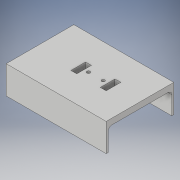
# Autodesk Inventor part: breadBoardMt
Saved by Autodesk Inventor 2019 (Build 230136000, 136)
## iProperties
Created: 2019-10-26
Part Number: breadBoardMt
Material: Generic
Document SubType Name: Modeling
Designer: test
Density: 1 g/cm^3
Appearance: Default
Author: test
Autodesk Inventor part; units mm, degrees
ref_plane "YZ Plane" through (0, 0, 0) normal (1, 0, 0) x (0, 1, 0)
ref_plane "XZ Plane" through (0, 0, 0) normal (0, 1, 0) x (-1, 0, 0)
ref_plane "XY Plane" through (0, 0, 0) normal (0, 0, 1) x (1, 0, 0)
sketch "Sketch1" plane through (0, 0, 0) normal (0, 1, 0) x (-1, 0, 0)
  line L0 (26.4284, 7.2103) -> (-59.9316, 7.2103)
  line L1 (-59.9316, 7.2103) -> (-59.9316, -51.2097)
  line L2 (-59.9316, -51.2097) -> (26.4284, -51.2097)
  line L3 (26.4284, -51.2097) -> (26.4284, 7.2103)
  point P0 (0, 0)
  dimension "d0" = 58.42
  dimension "d1" = 86.36
  constraints: 8 end point, 2 parallel, 1 horizontal, 1 perpendicular
  measures "d0" distance of L2.end L0.start
  measures "d1" distance of L1.end L2.end
extrude "Extrusion1" add sketch "Sketch1" along normal blind 12.7
sketch "Sketch9" plane through (0, 0, 0) normal (0, -1, 0) x (1, 0, 0)
  line L0 (-26.4284, 7.2103) -> (59.9316, 7.2103) projected
  line L1 (-26.4284, -51.2097) -> (-26.4284, 7.2103) projected
  line L2 (59.9316, -51.2097) -> (-26.4284, -51.2097) projected
  line L3 (59.9316, 7.2103) -> (59.9316, -51.2097) projected
  point P0 (0, 0)
extrude "Extrusion6" add sketch "Sketch9" along normal blind 5.08
ref_plane "Work Plane1" through (59.9316, 9.525, 7.2103) normal (1, 0, 0) x (0, 0, -1)
sketch "Sketch10" plane through (59.9316, 9.525, 7.2103) normal (1, 0, 0) x (0, 0, -1)
  line L0 (56.642, -10.795) -> (1.778, -10.795)
  line L1 (1.778, -10.795) -> (1.778, -0.635)
  line L2 (1.778, -0.635) -> (56.642, -0.635)
  line L3 (56.642, -0.635) -> (56.642, -10.795)
  line L4 (0, -14.605) -> (0, 3.175) projected
  line L5 (58.42, -14.605) -> (58.42, 3.175) projected
  line L6 (58.42, -14.605) -> (0, -14.605) projected
  dimension "d26" = 10.16
  dimension "d105" = 1.778
  dimension "d106" = 1.778
  dimension "d107" = 3.81
  constraints: 8 end point, 2 parallel, 1 horizontal, 1 perpendicular
  measures "d26" distance of L0.end L1.end
  measures "d105" distance between parallel lines of L4 L1
  measures "d106" distance between parallel lines of L5 L3
  measures "d107" distance between parallel lines of L6 L0
extrude "Extrusion7" cut sketch "Sketch10" against normal blind 82.55
sketch "Sketch12" plane through (0, -5.08, 0) normal (0, -1, 0) x (1, 0, 0)
  line L0 (53.3019, 5.4323) -> (59.9316, 5.4323)
  line L1 (59.9316, 5.4323) -> (59.9316, -49.4317)
  line L2 (59.9316, -49.4317) -> (53.3019, -49.4317)
  line L3 (53.3019, 5.4323) -> (2.5019, 5.4323)
  line L4 (2.5019, 5.4323) -> (2.5019, -49.4317)
  line L5 (2.5019, -49.4317) -> (53.3019, -49.4317)
  line L6 (59.9316, -49.4317) -> (59.9316, 5.4323) projected
  line L7 (59.9316, 5.4323) -> (2.5019, 5.4323)
  line L8 (2.5019, 5.4323) -> (2.5019, -49.4317)
  line L9 (2.5019, -49.4317) -> (59.9316, -49.4317)
  line L10 (59.9316, -49.4317) -> (59.9316, 5.4323)
  point P0 (0, 0)
  point P1 (59.9316, 5.4323)
  point P2 (-22.6184, -49.4317)
  constraints: 20 end point, 3 parallel, 3 perpendicular, 2 horizontal
extrude "Extrusion9" cut sketch "Sketch12" against normal blind 10.16
sketch "Sketch16" plane through (0, -5.08, 0) normal (0, -1, 0) x (1, 0, 0)
  line L0 (2.5019, -49.4317) -> (2.5019, 5.4323) projected
  line L1 (2.5019, -9.6861) -> (-5.864, -9.6861)
  line L2 (-5.864, -9.6861) -> (-5.864, -34.3133)
  line L3 (-5.864, -34.3133) -> (2.5019, -34.3133)
  line L4 (2.5019, -34.3133) -> (2.5019, -9.6861)
  point P0 (0, 0)
  constraints: 8 end point, 2 parallel, 1 horizontal, 1 perpendicular
extrude "Extrusion12" add sketch "Sketch16" against normal blind 3.81
fillet "Fillet7" radius 3.175 2 edges at (2.5019, -3.175, 5.4323) (2.5019, -3.175, -49.4317)
sketch "Sketch17" plane through (0, -5.08, 0) normal (0, -1, 0) x (1, 0, 0)
  line L0 (2.5019, -46.2567) -> (2.5019, 2.2573) projected
  arc A0 (5.6769, 5.4323) -> (2.5019, 2.2573) centre (5.6769, 2.2573) ccw projected
  line L1 (5.6769, 5.4323) -> (59.9316, 5.4323) projected
  line L2 (59.9316, 5.4323) -> (59.9316, 7.2103) projected
  line L3 (59.9316, 7.2103) -> (-26.4284, 7.2103) projected
  line L4 (-26.4284, 7.2103) -> (-26.4284, -51.2097) projected
  line L5 (-26.4284, -51.2097) -> (59.9316, -51.2097) projected
  line L6 (59.9316, -51.2097) -> (59.9316, -49.4317) projected
  line L7 (59.9316, -49.4317) -> (5.6769, -49.4317) projected
  arc A1 (2.5019, -46.2567) -> (5.6769, -49.4317) centre (5.6769, -46.2567) ccw projected
  point P0 (0, 0)
extrude "Extrusion13" add sketch "Sketch17" along normal blind 5.08
sketch "Sketch18" plane through (59.9316, 8.89, -49.4317) normal (0, -1, 0) x (1, 0, 0)
  line L0 (0, 54.864) -> (0, 0) projected
  line L1 (0, 54.864) -> (-82.55, 54.864) projected
  line L2 (-82.55, 54.864) -> (-82.55, 0) projected
  line L3 (0, 0) -> (-82.55, 0) projected
  point P0 (-59.9316, 49.4317)
extrude "Extrusion14" cut sketch "Sketch18" along normal blind 16.764
sketch "Sketch19" plane through (0, -10.16, 0) normal (0, -1, 0) x (1, 0, 0)
  line L0 (-2.4549, 1.4804) -> (-2.4549, -9.5517) construction
  line L1 (-2.4549, -9.5517) -> (-23.2018, -9.5517) construction
  line L2 (-23.2018, -9.5517) -> (-23.2018, 1.4804) construction
  line L3 (-23.2018, 1.4804) -> (-2.4549, 1.4804) construction
  line L4 (-12.7853, 0.4272) -> (-2.6253, 0.4272)
  line L5 (-2.6253, 0.4272) -> (-2.6253, -1.563)
  line L6 (-2.6253, -1.563) -> (-9.4399, -5.7369)
  line L7 (-9.4399, -5.7369) -> (-2.6253, -5.7369)
  line L8 (-2.6253, -5.7369) -> (-2.6253, -7.6342)
  line L9 (-2.6253, -7.6342) -> (-12.7853, -7.6342)
  line L10 (-12.7853, -7.6342) -> (-12.7853, -5.582)
  line L11 (-12.7853, -5.582) -> (-6.1178, -1.47)
  line L12 (-6.1178, -1.47) -> (-12.7853, -1.47)
  line L13 (-12.7853, -1.47) -> (-12.7853, 0.4272)
  line L14 (-9.4709, -13.2253) -> (-9.2773, -15.2232)
  spline S0 degree 2 poles (-9.2773, -15.2232) (-10.284, -15.4013) (-11.2287, -16.5087) (-11.2287, -17.438) knots 0 0 0 1 2 2 2
  spline S1 degree 2 poles (-11.2287, -17.438) (-11.2287, -18.4292) (-10.3924, -19.4359) (-9.8271, -19.4359) knots 0 0 0 1 2 2 2
  spline S2 degree 2 poles (-9.8271, -19.4359) (-9.4631, -19.4359) (-8.9598, -19.01) (-8.7739, -18.4834) knots 0 0 0 1 2 2 2
  spline S3 degree 2 poles (-8.7739, -18.4834) (-8.65, -18.1272) (-8.3325, -16.8417) knots 0 0 0 1 1 1
  spline S4 degree 2 poles (-8.3325, -16.8417) (-7.9221, -15.1922) (-7.3258, -14.5262) knots 0 0 0 1 1 1
  spline S5 degree 2 poles (-7.3258, -14.5262) (-6.4895, -13.5892) (-5.2892, -13.5892) knots 0 0 0 1 1 1
  spline S6 degree 2 poles (-5.2892, -13.5892) (-4.507, -13.5892) (-3.1596, -14.472) (-2.4549, -16.1292) (-2.4549, -17.2986) knots 0 0 0 1 2 3 3 3
  spline S7 degree 2 poles (-2.4549, -17.2986) (-2.4549, -19.2113) (-4.1276, -21.1473) (-5.5292, -21.1937) knots 0 0 0 1 2 2 2
  line L15 (-5.5292, -21.1937) -> (-5.6222, -19.1416)
  spline S8 degree 2 poles (-5.6222, -19.1416) (-4.84, -19.01) (-4.1508, -18.1426) (-4.1508, -17.2753) knots 0 0 0 1 2 2 2
  spline S9 degree 2 poles (-4.1508, -17.2753) (-4.1508, -16.377) (-4.5148, -15.8737) knots 0 0 0 1 1 1
  spline S10 degree 2 poles (-4.5148, -15.8737) (-4.7548, -15.5484) (-5.1498, -15.5484) knots 0 0 0 1 1 1
  spline S11 degree 2 poles (-5.1498, -15.5484) (-5.506, -15.5484) (-5.7693, -15.8505) knots 0 0 0 1 1 1
  spline S12 degree 2 poles (-5.7693, -15.8505) (-6.0945, -16.2454) (-6.7992, -19.2423) (-7.5504, -20.6749) (-8.8591, -21.488) (-9.8271, -21.488) knots 0 0 0 1 2 3 4 4 4
  spline S13 degree 2 poles (-9.8271, -21.488) (-10.6944, -21.488) (-12.22, -20.52) (-12.9634, -18.7467) (-12.9634, -17.4225) knots 0 0 0 1 2 3 3 3
  spline S14 degree 2 poles (-12.9634, -17.4225) (-12.9634, -15.4942) (-11.1823, -13.4266) (-9.4709, -13.2253) knots 0 0 0 1 2 2 2
  line L16 (-12.7853, -27.0946) -> (-2.6253, -27.0946)
  line L17 (-2.6253, -27.0946) -> (-2.6253, -29.1467)
  line L18 (-2.6253, -29.1467) -> (-12.7853, -29.1467)
  line L19 (-12.7853, -29.1467) -> (-12.7853, -27.0946)
  line L20 (-12.7853, -35.0631) -> (-2.6253, -35.0631)
  line L21 (-2.6253, -35.0631) -> (-2.6253, -37.0533)
  line L22 (-2.6253, -37.0533) -> (-9.4399, -41.2272)
  line L23 (-9.4399, -41.2272) -> (-2.6253, -41.2272)
  line L24 (-2.6253, -41.2272) -> (-2.6253, -43.1245)
  line L25 (-2.6253, -43.1245) -> (-12.7853, -43.1245)
  line L26 (-12.7853, -43.1245) -> (-12.7853, -41.0723)
  line L27 (-12.7853, -41.0723) -> (-6.1178, -36.9603)
  line L28 (-6.1178, -36.9603) -> (-12.7853, -36.9603)
  line L29 (-12.7853, -36.9603) -> (-12.7853, -35.0631)
  point P0 (0, 0)
  constraints: 2 other
emboss "Emboss2" sketch "Sketch19" operation add depth 1.27 direction (0, 1, 0)
ref_plane "Work Plane2" through (-26.4284, 9.525, -51.2097) normal (-1, 0, 0) x (0, 0, 1)
sketch "Sketch20" plane through (-26.4284, 9.525, -51.2097) normal (-1, 0, 0) x (0, 0, 1)
  line L0 (0, -19.685) -> (0, 0) construction
  line L1 (0, -19.685) -> (0, 3.175) construction
  line L2 (58.42, -19.685) -> (0, -19.685) construction
  line L3 (58.42, 3.175) -> (58.42, -19.685) construction
  line L4 (58.42, -10.795) -> (0, -10.795) construction
  line L5 (34.925, -19.685) -> (23.495, -19.685)
  line L6 (23.495, -19.685) -> (23.495, -12.065)
  line L7 (23.495, -12.065) -> (34.925, -12.065)
  line L8 (34.925, -12.065) -> (34.925, -19.685)
  line L9 (0, 3.175) -> (58.42, 3.175) projected
  point P0 (58.42, 0)
  point P1 (29.21, -19.685)
  dimension "d77" = 7.62
  dimension "d104" = 11.43
  constraints: 10 end point, 2 horizontal, 2 midpoint, 2 parallel, 2 point on line, 1 perpendicular
  measures "d77" distance of L5.end L6.end
  measures "d104" distance between parallel lines of L8 L6
extrude "Extrusion15" cut sketch "Sketch20" against normal blind 5.08
sketch "Sketch21" plane through (0, 12.7, 0) normal (0, 1, 0) x (1, 0, 0)
  point P0 (0, 0)
sketch "Sketch22" plane through (0, 12.7, 0) normal (0, 1, 0) x (1, 0, 0)
  line L0 (-26.4284, -7.2103) -> (59.9316, -7.2103) projected
  line L1 (59.9316, -7.2103) -> (59.9316, 51.2097) projected
  line L2 (59.9316, 51.2097) -> (-26.4284, 51.2097) projected
  line L3 (-26.4284, 51.2097) -> (-26.4284, -7.2103) projected
  point P0 (0, 0)
extrude "Extrusion16" add sketch "Sketch22" along normal blind 1.27
fillet "Fillet10" radius 3.175 2 edges at (18.6566, 8.89, 5.4323) (18.6566, 8.89, -49.4317)
sketch "Sketch23" plane through (0, 13.97, 0) normal (0, 1, 0) x (1, 0, 0)
  line L0 (-26.4284, 51.2097) -> (59.9316, 51.2097) projected
  line L1 (16.7516, 51.2097) -> (16.7516, 43.4082)
  line L2 (31.9916, 28.3497) -> (37.0716, 28.3497)
  line L3 (37.0716, 28.3497) -> (37.0716, 15.6497)
  line L4 (37.0716, 15.6497) -> (31.9916, 15.6497)
  line L5 (31.9916, 15.6497) -> (31.9916, 28.3497)
  line L6 (31.9916, 28.3497) -> (37.0716, 15.6497) construction
  line L7 (37.0716, 28.3497) -> (31.9916, 15.6497) construction
  line L8 (34.5316, 51.2097) -> (34.5316, -7.2103) construction
  line L9 (59.9316, -7.2103) -> (-26.4284, -7.2103) construction
  line L10 (59.9316, -7.2103) -> (59.9316, 51.2097) construction
  line L11 (9.1316, 51.2097) -> (9.1316, -7.2103) construction
  line L12 (6.5916, 28.3497) -> (11.6716, 28.3497)
  line L13 (11.6716, 28.3497) -> (11.6716, 15.6497)
  line L14 (11.6716, 15.6497) -> (6.5916, 15.6497)
  line L15 (6.5916, 15.6497) -> (6.5916, 28.3497)
  line L16 (6.5916, 28.3497) -> (11.6716, 15.6497) construction
  line L17 (11.6716, 28.3497) -> (6.5916, 15.6497) construction
  line L18 (34.5316, 21.9997) -> (9.1316, 21.9997) construction
  circle A0 centre (28.1816, 21.9997) radius 1.3891
  circle A1 centre (15.4816, 21.9997) radius 1.3891
  point P0 (34.5316, 21.9997)
  point P1 (9.1316, 21.9997)
  point P2 (21.8316, 21.9997)
  dimension "d89" = 12.7
  dimension "d90" = 5.08
  dimension "d91" = 25.4
  dimension "d94" = 25.4
  dimension "d101" = 2.7781
  dimension "d102" = 6.35
  dimension "d103" = 6.35
  constraints: 32 end point, 8 midpoint, 4 point on line, 3 horizontal, 2 centre point, 2 parallel, 2 vertical, 1 equal radius, 1 perpendicular, 15 other
  measures "d89" distance of L2.end L3.end
  measures "d90" distance of L3.end L4.end
  measures "d91" distance between parallel lines of L10 L8
  measures "d94" distance of L8.start L11.start
  measures "d101" diameter of A0
  measures "d102" distance of A0.centre point (21.832, 22)
  measures "d103" distance of A1.centre point (21.832, 22)
extrude "Extrusion17" cut sketch "Sketch23" against normal through all
equation "\"d106\" = d105"
equation "\"d103\" = d102"
body "Solid1"
